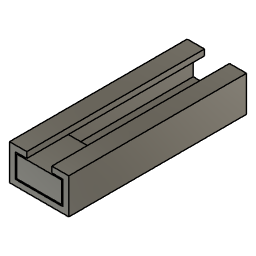
Slider Joint Trial (Autodesk Fusion 360 design; units mm, degrees)
Autodesk Fusion 360 part; units mm, degrees
sketch "Sketch4" plane through (0, 0, 0) normal (0, 0, 1) x (1, 0, 0)
  line L0 (0, 0) -> (-250, 0)
  line L1 (-250, 0) -> (-250, 750)
  line L2 (-250, 750) -> (0, 750)
  line L3 (0, 750) -> (0, 0)
  constraint horizontal L0
  constraint vertical L1
  constraint horizontal L2
  constraint vertical L3
  constraint coincident L0.start L3.end
extrude "Extrude1" add sketch "Sketch4" along normal blind 150 makes body 1
sketch "Sketch5" plane through (0, 0, 0) normal (0, -1, 0) x (1, 0, 0)
  line L0 (-250, 0) -> (0, 0)
  line L1 (0, 0) -> (0, 150)
  line L2 (0, 150) -> (-250, 150)
  line L3 (-250, 150) -> (-250, 0)
  line L4 (-225, 125) -> (-25, 125)
  line L5 (-25, 125) -> (-25, 25)
  line L6 (-25, 25) -> (-225, 25)
  line L7 (-225, 25) -> (-225, 125)
  constraint horizontal L4
  constraint vertical L5
  constraint horizontal L6
  constraint vertical L7
extrude "Extrude2" cut sketch "Sketch5" against normal blind 850 contours L4 L5 L6 L7 bodies 1
sketch "Sketch6" plane through (0, 0, 150) normal (0, 0, 1) x (-1, 0, 0)
  line L0 (0, -750) -> (250, -750)
  line L1 (250, -750) -> (250, 0)
  line L2 (250, 0) -> (0, 0)
  line L3 (0, 0) -> (0, -750)
  line L4 (177.2752, -750) -> (71.4878, -750)
  line L5 (71.4878, -750) -> (71.4878, 0)
  line L6 (71.4878, 0) -> (177.2752, 0)
  line L7 (177.2752, 0) -> (177.2752, -750)
  constraint horizontal L4
  constraint vertical L5
  constraint horizontal L6
  constraint vertical L7
  constraint coincident L2 L5.end
  constraint coincident L0 L4.start
extrude "Extrude3" cut sketch "Sketch6" against normal blind 50 contours L0 L2 L4 L5 L6 L7 bodies 1
sketch "Sketch7" plane through (0, 0, 0) normal (0, -1, 0) x (1, 0, 0)
  line L0 (-177.2752, 125) -> (-177.2752, 150)
  line L1 (-177.2752, 150) -> (-250, 150)
  line L2 (-250, 150) -> (-250, 0)
  line L3 (-250, 0) -> (0, 0)
  line L4 (0, 0) -> (0, 150)
  line L5 (0, 150) -> (-71.4878, 150)
  line L6 (-71.4878, 150) -> (-71.4878, 125)
  line L7 (-71.4878, 125) -> (-25, 125)
  line L8 (-25, 125) -> (-25, 25)
  line L9 (-25, 25) -> (-225, 25)
  line L10 (-225, 25) -> (-225, 125)
  line L11 (-225, 125) -> (-177.2752, 125)
  line L12 (-220, 120) -> (-30, 120)
  line L13 (-30, 120) -> (-30, 30)
  line L14 (-30, 30) -> (-220, 30)
  line L15 (-220, 30) -> (-220, 120)
  constraint horizontal L12
  constraint vertical L13
  constraint horizontal L14
  constraint vertical L15
extrude "Extrude4" add sketch "Sketch7" against normal blind 180 separate body contours L12 L13 L14 L15 makes body 2
copy_body "Body->Comp1" bodies 1 removing the originals makes body 3 in component "Component"
copy_body "Body->Comp2" bodies 2 removing the originals makes body 4 in component "Component'"
component "Component" placed x (1, 0, 0) y (0, 1, 0) z (0, 0, 1) at (0, 0, 0)
component "Component'" placed x (1, 0, 0) y (0, 1, 0) z (0, 0, 1) at (0, 0, 0)
